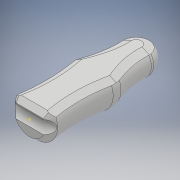
# Autodesk Inventor part: Finger_small
Saved by Autodesk Inventor 2017 (Build 210142000, 142)
## iProperties
Created: 2016-12-17
Part Number: Finger_small
Material: Generic
Document SubType Name: Modeling
Designer: Samanth
Density: 1 g/cm^3
Appearance: Default
Author: Samanth
Autodesk Inventor part; units mm, degrees
ref_plane "YZ Plane" through (0, 0, 0) normal (1, 0, 0) x (0, 1, 0)
ref_plane "XZ Plane" through (0, 0, 0) normal (0, 1, 0) x (-1, 0, 0)
ref_plane "XY Plane" through (0, 0, 0) normal (0, 0, 1) x (1, 0, 0)
sketch "Sketch1" plane through (0, 0, 0) normal (0, 0, 1) x (1, 0, 0)
  line L0 (0, 0) -> (10, 0)
  line L1 (0, 30) -> (0, 0)
  line L2 (0, 55) -> (0, 30)
  arc A0 (10, 30) -> (10, 0) centre (90.5968, 15) ccw
  line L3 (0, 55) -> (7, 55)
  line L4 (7, 48.1794) -> (7, 55)
  arc A1 (7, 48.1794) -> (10, 30) centre (51.1431, 46.1267) ccw
  dimension "d5" = 7
  constraints: 10 end point, 4 point on circle, 2 centre point, 2 horizontal, 1 collinear, 1 perpendicular, 1 point on line
  measures "d5" distance of L2.start L3.end
revolve "Revolution1" add sketch "Sketch1" angle 360 about axis through (0, 55, 0) along (0, -1, 0)
fillet "Fillet1" radius 7 1 edges at (-7, 55, 0)
sketch "Sketch2" plane through (0, 0, 0) normal (1, 0, 0) x (0, 1, 0)
  point P0 (0, 0)
sketch "Sketch3" plane through (0, 0, 0) normal (1, 0, 0) x (0, 1, 0)
  circle A0 centre (0, 0) radius 2.925
  dimension "d7" = 5.85
  constraints: 1 centre point, 1 coincident
  measures "d7" diameter of A0
extrude "Extrusion1" cut sketch "Sketch3" along normal mid plane 25
sketch "Sketch4" plane through (0, 0, 0) normal (0, -1, 0) x (1, 0, 0)
  point P0 (0, 0)
sketch "Sketch5" plane through (0, 0, 0) normal (0, -1, 0) x (1, 0, 0)
  circle A0 centre (0, 0) radius 10 projected
  line L0 (-8.4117, 5.4078) -> (8.4117, 5.4078)
  arc A1 (8.4117, 5.4078) -> (-8.4117, 5.4078) centre (0, 0) ccw
  constraints: 4 point on circle, 2 end point, 1 centre point, 1 horizontal
extrude "Extrusion2" cut sketch "Sketch5" against normal blind 60 contours L0 A0 picked at (-2.2711, 6.0451)
chamfer "Chamfer1" distance 2 angle 45 5 edges at (6.7076, 15, 5.4078) (-6.7076, 15, 5.4078) (5.2809, 38.8319, 5.4078) (-5.2809, 38.8319, 5.4078) (0, 52.4448, 5.4078)
fillet "Fillet2" radius 8 1 edges at (0, 30, -10)
fillet "Fillet3" radius 6 2 edges at (6.688, 48.1463, 2.0614) (-2.0614, 48.1463, -6.688)
chamfer "Chamfer2" distance 2.1 angle 45 1 edges at (0, 0, 5.4078)
chamfer "Chamfer3" distance 3.1 angle 45 1 edges at (0, 0, -10)
body "Solid1"
